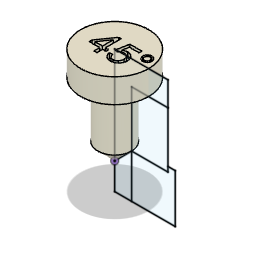
electrode punch tool v16 (Autodesk Fusion 360 design; units mm, degrees)
Autodesk Fusion 360 part; units mm, degrees
sketch "Sketch1" plane through (0, 0, 0) normal (0, 0, 1) x (1, 0, 0)
  line L0 (0, 0) -> (3.5, 3.5)
  line L1 (3.5, 3.5) -> (3.5, 15)
  line L2 (3.5, 15) -> (11, 15)
  line L3 (11, 15) -> (11, 20)
  line L4 (11, 20) -> (0, 20)
  line L5 (0, 20) -> (0, 0)
  line L6 (0.025, 0.025) -> (0, 0.025)
  line L7 (3.5, 3.5) -> (11, 3.5)
  line L8 (11, 3.5) -> (11, 15)
  line L9 (12.5, 4.5) -> (12.5, -5.5)
  line L10 (12.5, -5.5) -> (0, -5.5)
  line L11 (0, -5.5) -> (0, 0)
  line L12 (12.5, 4.5) -> (11, 4.5)
  line L13 (3.5, 3.5) -> (3.5, -5.5)
  dimension "d1" = 45
  dimension "d2" = 3.5
  dimension "d3" = 15
  dimension "d4" = 5
  dimension "d5" = 11
  dimension "d7" = 0.025
  dimension "d8" = 12.5
  dimension "d9" = 1
  dimension "d10" = 10
  constraint coincident L0.start L5.end
  constraint vertical L1
  constraint perpendicular L1 L2
  constraint perpendicular L2 L3
  constraint perpendicular L3 L4
  constraint perpendicular L4 L5
  constraint coincident L0 L6.start
  constraint coincident L5 L6.end
  constraint perpendicular L5 L6
  constraint perpendicular L1 L7
  constraint vertical L8
  constraint vertical L9
  constraint perpendicular L9 L10
  constraint perpendicular L10 L11
  constraint coincident L8 L12.end
  constraint perpendicular L8 L12
  constraint coincident L10 L13.end
  constraint perpendicular L10 L13
  measures "d1" angle of L0 L5
  measures "d2" distance of L1 L5
  measures "d3" distance of L0.start L2
  measures "d4" distance of L2.end L3.end
  measures "d5" distance of L3.end L4.end
  measures "d7" distance of L6.start L6.end
  measures "d8" distance of L9.end L10.end
  measures "d9" distance of L7 L12
  measures "d10" distance of L9.start L9.end
revolve "Revolve1" add sketch "Sketch1" angle 360 about axis through (0, 20, 0) along (0, -1, 0) contours L0 L1 L2 L3 L4 L5 L6 makes body 1
revolve "Revolve2" add sketch "Sketch1" angle 360 about axis through (0, 3.5, 0) along (0, 1, 0) separate body contours L1 L2 L7 L8 makes body 2
revolve "Revolve3" add sketch "Sketch1" angle 360 about axis through (0, 3.5, 0) along (0, 1, 0) separate body contours L7 L8 L9 L10 L12 L13 makes body 3
move_face "OffsetFaces1" offset -0.1 1 faces at (3.4956, 7.3333, 0.1745) on bodies 2
move_face "OffsetFaces2" offset -0.3 1 faces at (3.4826, -2.5, 0.3485) on bodies 3
move_face "OffsetFaces3" offset -0.3 1 faces at (10.9863, 4.1667, 0.5483) on bodies 3
move_face "OffsetFaces4" offset -4 1 faces at (10.9863, 16.6667, -0.5483) on bodies 1
copy_body "Body->Comp1" bodies 1 removing the originals makes body 4 in component "punch"
copy_body "Body->Comp2" bodies 2 removing the originals makes body 5 in component "guide"
copy_body "Body->Comp3" bodies 3 removing the originals makes body 6 in component "die"
sketch "Skizze2" plane through (0, 20, 0) normal (0, 1, 0) x (-1, 0, 0)
  circle A0 centre (0, 0) radius 7
  line L0 (3.9919, 2.5123) -> (-3.9868, 2.5203) construction
  line L1 (-3.9868, 2.5203) -> (-3.9919, -2.5123) construction
  line L2 (-3.9919, -2.5123) -> (3.9868, -2.5203) construction
  line L3 (3.9868, -2.5203) -> (3.9919, 2.5123) construction
  dimension "d18" = 5
  text T0 "45°" font "Arial" height 5 align left top in box 7.9787 x 5.0326 at (3.9919, 2.5123) x (-0.999999, 0.00101) y (-0.00101, -0.999999) spacing 1
  constraint coincident A0.centre
extrude "Extrusion1" cut sketch "Skizze2" against normal blind 1 text T0 bodies 4 in component "punch"
component "punch" placed x (1, 0, 0) y (0, 1, 0) z (0, 0, 1) at (0, 0, 0)
component "guide" placed x (1, 0, 0) y (0, 1, 0) z (0, 0, 1) at (0, 0, 0)
component "die" placed x (1, 0, 0) y (0, 1, 0) z (0, 0, 1) at (0, 0, 0)
named bodies: "punch", "guide", "die"
